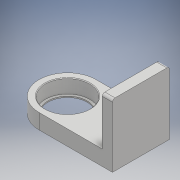
# Autodesk Inventor part: Porta cuscinetto perno telaietto
Saved by Autodesk Inventor 2018 (Build 220112000, 112)
## iProperties
Created: 2020-06-11
Part Number: Porta cuscinetto perno telaietto
Material: Generico
Document SubType Name: Modeling
Designer: Francesco
Density: 1 g/cm^3
Appearance: Default
Author: Francesco
Autodesk Inventor part; units mm, degrees
ref_plane "YZ Plane" through (0, 0, 0) normal (1, 0, 0) x (0, 1, 0)
ref_plane "XZ Plane" through (0, 0, 0) normal (0, 1, 0) x (-1, 0, 0)
ref_plane "XY Plane" through (0, 0, 0) normal (0, 0, 1) x (1, 0, 0)
sketch "Schizzo1" plane through (0, 0, 0) normal (0, 0, 1) x (1, 0, 0)
  arc A0 (0, 22.5) -> (0, -22.5) centre (0, 0) ccw
  line L0 (0, 22.5) -> (50, 22.5)
  line L1 (50, 22.5) -> (50, -22.5)
  line L2 (50, -22.5) -> (0, -22.5)
  dimension "d1" = 45
  dimension "d2" = 50
  constraints: 6 end point, 2 perpendicular, 2 point on circle, 1 centre point, 1 horizontal, 1 tangent
  measures "d1" diameter of A0
  measures "d2" distance of L0.start L0.end
extrude "Estrusione1" add sketch "Schizzo1" along normal blind 12
sketch "Schizzo2" plane through (0, 0, 12) normal (0, 0, 1) x (1, 0, 0)
  circle A0 centre (0, 0) radius 17.5
  dimension "d5" = 35
  constraints: 1 centre point, 1 coincident
  measures "d5" diameter of A0
extrude "Estrusione2" cut sketch "Schizzo2" against normal blind 11
sketch "Schizzo3" plane through (0, 0, 1) normal (0, 0, 1) x (1, 0, 0)
  circle A0 centre (0, 0) radius 15.5
  dimension "d8" = 31
  constraints: 1 centre point, 1 coincident
  measures "d8" diameter of A0
extrude "Estrusione3" cut sketch "Schizzo3" against normal up to next
chamfer "Smusso1" distance 0.5 angle 45 1 edges at (-17.5, 0, 12)
sketch "Schizzo4" plane through (50, -22.5, 0) normal (1, 0, 0) x (0, 0, -1)
  line L0 (0, 45) -> (0, 0) projected
  line L1 (0, 45) -> (-50, 45)
  line L2 (-50, 45) -> (-50, 0)
  line L3 (-50, 0) -> (0, 0)
  line L4 (0, 0) -> (0, 45)
  point P0 (0, 22.5)
  dimension "d15" = 50
  dimension "d16" = 45
  constraints: 8 end point, 2 parallel, 1 horizontal, 1 perpendicular
  measures "d15" distance of L3.end L2.end
  measures "d16" distance of L2.end L1.end
extrude "Estrusione4" add sketch "Schizzo4" along normal blind 8
fillet "Raccordo2" radius 2 2 edges at (54, 22.5, 50) (54, -22.5, 50)
